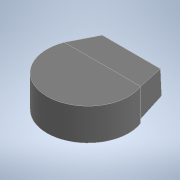
# Autodesk Inventor part: vez-nova
Saved by Autodesk Inventor 2022 (Build 260153000, 153)
## iProperties
Created: 2022-12-19
Part Number: vez-nova
Material: Generic
Document SubType Name: Modeling
Designer: matys
Density: 1 g/cm^3
Appearance: Gray
Author: matys
Autodesk Inventor part; units mm, degrees
ref_plane "YZ Plane" through (0, 0, 0) normal (1, 0, 0) x (0, 1, 0)
ref_plane "XZ Plane" through (0, 0, 0) normal (0, 1, 0) x (-1, 0, 0)
ref_plane "XY Plane" through (0, 0, 0) normal (0, 0, 1) x (1, 0, 0)
sketch "Sketch1" plane through (0, 0, 0) normal (0, 1, 0) x (-1, 0, 0)
  arc A0 (46.7052, -17.85) -> (-46.7052, -17.85) centre (0, 0) ccw
  line L0 (0, 0) -> (0, -55.2)
  line L1 (0, -55.2) -> (35, -55.2)
  line L2 (0, -55.2) -> (-35, -55.2)
  line L3 (0, 50) -> (0, -17.85)
  line L4 (0, -17.85) -> (46.7052, -17.85)
  line L5 (0, -17.85) -> (-46.7052, -17.85)
  line L6 (-46.7052, -17.85) -> (-35, -55.2)
  line L7 (46.7052, -17.85) -> (35, -55.2)
  line L8 (35, -55.2) -> (33, -55.2)
  line L9 (-35, -55.2) -> (-33, -55.2)
  line L10 (0, 50) -> (0, 48)
  arc A1 (44.5576, -17.85) -> (-44.5576, -17.85) centre (0, 0) ccw
  line L11 (44.5576, -17.85) -> (33, -55.2)
  line L12 (-44.5576, -17.85) -> (-33, -55.2)
  dimension "d0" = 100
  dimension "d4" = 55.2
  dimension "d5" = 35
  dimension "d6" = 67.85
  dimension "d7" = 2
  dimension "d8" = 2
  dimension "d9" = 2
  constraints: 26 end point, 7 point on line, 6 point on circle, 3 coincident, 2 centre point, 1 horizontal, 1 perpendicular
  measures "d0" diameter of A0
  measures "d4" distance of L0.start L0.end
  measures "d5" distance of L0.end L2.end
  measures "d6" distance of L3.start L3.end
  measures "d7" distance of L1.end L8.end
  measures "d8" distance of L2.end L9.end
  measures "d9" distance of L3.start L10.end
extrude "Extrusion1" add sketch "Sketch1" along normal blind 34.5
chamfer "Chamfer3" distance 2.3 distance2 34.5 2 edges at (-17.5, 34.5, -55.2) (17.5, 34.5, -55.2) measured on face at (-17.5, 34.5, -54.7) measured on face at (17.5, 34.5, -54.7)
chamfer "Chamfer4" distance 4.6 distance2 35.05 2 edges at (-17.8604, 34.5, -52.9001) (17.8604, 34.5, -52.9001) measured on face at (17.8604, 34.0011, -52.9334) measured on face at (-17.8604, 34.0011, -52.9334)
sketch "Sketch3" plane through (0, 0, 0) normal (0, -1, 0) x (1, 0, 0)
  line L0 (0, 0) -> (0, 34.5)
  circle A0 centre (0, 0) radius 34.5
  circle A1 centre (0, 0) radius 36.8
  circle A2 centre (0, 0) radius 37.375
  line L1 (0, -36.8) -> (0, -41.4)
  line L2 (0, -41.4) -> (17.5375, -41.4)
  line L3 (0, -41.4) -> (-17.5375, -41.4)
  arc A3 (46.7052, -17.85) -> (-46.7052, -17.85) centre (0, 0) ccw
  line L4 (46.7052, -17.85) -> (35, -55.2) projected
  line L5 (46.7052, -17.85) -> (17.5375, -41.4)
  arc A4 (46.7052, -17.85) -> (-46.7052, -17.85) centre (0, 0) ccw projected
  line L6 (-46.7052, -17.85) -> (-17.5375, -41.4)
  dimension "d25" = 73.6
  dimension "d24" = 34.5
  dimension "d26" = 74.75
  dimension "d27" = 4.6
  dimension "d28" = 17.5375
  constraints: 12 end point, 4 coincident, 2 centre point, 2 point on circle, 2 vertical, 2 vertical alignment, 1 horizontal, 1 symmetric about line, 4 other
  measures "d24" distance of L0.start L0.end
  measures "d26" diameter of A2
  measures "d27" distance of L1.start L1.end
  measures "d28" distance of L1.end L2.end
extrude "Extrusion2" add sketch "Sketch3" along normal blind 4.6 contours A0 | A1 | A2 | L3 L6 A3 L5 L2
sketch "Sketch4" plane through (0, -4.6, 0) normal (0, -1, 0) x (1, 0, 0)
  line L0 (0, 0) -> (0, -34.5)
  circle A0 centre (0, 0) radius 34.5
  line L1 (0, -34.5) -> (0, -37)
  circle A1 centre (0, 0) radius 37
  dimension "d31" = 34.5
  dimension "d32" = 2.5
  constraints: 4 end point, 2 coincident, 2 vertical, 2 vertical alignment, 4 other
  measures "d31" distance of L0.start L0.end
  measures "d32" distance of L0.end L1.end
extrude "Extrusion3" add sketch "Sketch4" along normal blind 5.75
sketch "Sketch5" plane through (0, -4.6, 0) normal (0, -1, 0) x (1, 0, 0)
  circle A0 centre (0, 0) radius 30.8955
  circle A1 centre (0, 0) radius 30
  dimension "d62" = 60
  constraints: 2 centre point, 2 coincident
  measures "d62" diameter of A1
extrude "Extrusion4" cut sketch "Sketch5" against normal blind 34.5 contours A1
sketch "Sketch6" plane through (0, -10.35, 0) normal (0, -1, 0) x (1, 0, 0)
  circle A0 centre (0, 0) radius 37
  constraints: 1 centre point, 1 coincident
extrude "Extrusion5" cut sketch "Sketch6" against normal blind 5.75
sketch "Sketch7" plane through (0, -4.6, 0) normal (0, -1, 0) x (1, 0, 0)
  line L0 (17.5375, -41.4) -> (-17.5375, -41.4) projected
  circle A0 centre (0, 0) radius 33.6
  circle A1 centre (0, 0) radius 30.0896
  dimension "d61" = 67.2
  constraints: 2 centre point, 1 coincident
  measures "d61" diameter of A0
extrude "Extrusion6" cut sketch "Sketch7" against normal blind 5.75 contours A0 | A1
sketch "Sketch8" plane through (0, 1.15, 0) normal (0, -1, 0) x (1, 0, 0)
  circle A0 centre (0, 0) radius 34.3955 projected
  line L0 (34.3955, 0) -> (-34.3955, 0)
  line L1 (41.6045, -3) -> (-34.3955, -3)
  line L2 (41.6045, 3) -> (-34.3955, 3)
  circle A1 centre (0, 0) radius 34.5
  circle A2 centre (0, 0) radius 34.3955
  circle A3 centre (0, 0) radius 30
  circle A4 centre (0, 0) radius 33.6
  point P0 (-34.3693, -3)
  point P1 (-34.3693, 3)
  point P2 (-34.2644, 3)
  point P3 (-34.2644, -3)
  point P4 (34.3693, -3)
  point P5 (34.2644, -3)
  point P6 (34.2644, 3)
  point P7 (34.3693, 3)
  point P8 (29.8496, -3)
  point P9 (29.8496, 3)
  point P10 (-29.8496, -3)
  point P11 (-29.8496, 3)
  point P12 (-33.4658, 3)
  point P13 (-33.4658, -3)
  point P14 (33.4658, -3)
  point P15 (33.4658, 3)
  dimension "d42" = 3
  dimension "d43" = 3
  constraints: 6 end point, 3 centre point, 3 coincident, 2 parallel, 2 point on circle, 1 horizontal, 1 horizontal alignment, 2 other
  measures "d42" distance between parallel lines of L0 L1
  measures "d43" distance between parallel lines of L0 L2
extrude "Extrusion7" cut sketch "Sketch8" against normal blind 5.75 contours A4 L1 A3 L0 | L0 A3 L2 A4 | L2 A3 L0 A4 | A4 L0 A3 L1
ref_plane "Work Plane1" through (8.75, 34.5, -17.85) normal (0, 0, 1) x (1, 0, 0)
sketch "Sketch9" plane through (8.75, 34.5, -17.85) normal (0, 0, 1) x (1, 0, 0)
  line L0 (37.9552, 0) -> (26.8749, -4.5898) projected
  line L1 (26.8749, -4.5898) -> (26.1514, -34.5)
  line L2 (37.9552, -34.5) -> (8.7875, -34.5) projected
  line L3 (-43.75, -34.5) -> (-44.3749, -4.5898) projected
  line L4 (-43.75, -34.5) -> (-40.75, -34.5)
  line L5 (-26.2875, -34.5) -> (-55.4552, -34.5) projected
  line L6 (-40.75, -34.5) -> (-40.75, -31.5)
  line L7 (-40.75, -31.5) -> (-40.75, -4.5898)
  line L8 (-40.75, -4.5898) -> (-40.75, -7.5898)
  line L9 (-40.75, -7.5898) -> (-40.75, -31.5)
  line L10 (25.75, -27.6) -> (25.75, -4.6) projected
  line L11 (26.8749, -4.5898) -> (26.25, -34.5) projected
  line L12 (26.25, -34.5) -> (23.25, -34.5)
  line L13 (23.25, -34.5) -> (23.25, -31.5)
  line L14 (23.25, -31.5) -> (-40.75, -31.5)
  line L15 (23.25, -31.5) -> (23.25, -7.5898)
  line L16 (23.25, -7.5898) -> (-40.75, -7.5898)
  point P0 (-8.75, -34.5)
  dimension "d46" = 3
  dimension "d47" = 3
  dimension "d48" = 3
  dimension "d49" = 3
  dimension "d50" = 3
  constraints: 22 end point, 6 point on line, 3 perpendicular, 1 parallel
  measures "d46" distance of L3.start L4.end
  measures "d47" distance of L4.end L6.end
  measures "d48" distance of L7.end L8.end
  measures "d49" distance of L11.end L12.end
  measures "d50" distance of L12.end L13.end
extrude "Extrusion8" cut sketch "Sketch9" along normal blind 10 and the other way blind 100 contours L7 L16 L15 L14
sketch "Sketch10" plane through (32, 3, -12.8938) normal (-1, 0, 0) x (0, 0, 1)
  line L0 (-42.1062, 0) -> (-40.5122, 23.9102)
  line L1 (-40.5122, 23.9102) -> (-41.3092, 11.9551)
  line L2 (-42.1062, 0) -> (-40.5122, 23.9102) projected
  line L3 (-41.3092, 11.9551) -> (-31.3092, 11.9551)
  line L4 (-31.3092, 11.9551) -> (-35.8092, 11.9551)
  circle A0 centre (-31.3092, 11.9551) radius 4.5
  point P0 (12.8938, -3)
  dimension "d55" = 10
  dimension "d56" = 4.5
  constraints: 8 end point, 1 coincident, 1 horizontal, 1 horizontal alignment, 1 midpoint, 1 point on line, 2 other
  measures "d55" distance of L1.end L3.end
  measures "d56" distance of L3.end L4.end
extrude "Extrusion9" cut sketch "Sketch10" along normal blind 66 and the other way blind 2
sketch "Sketch13" plane through (0, 29.9, 0) normal (0, -1, 0) x (1, 0, 0)
  line L0 (0, 0) -> (5.6, 0)
  line L1 (5.6, 0) -> (5.6, -5.6)
  line L2 (5.6, -5.6) -> (-5.6, -5.6)
  line L3 (-5.6, -5.6) -> (-5.6, 5.6)
  line L4 (-5.6, 5.6) -> (5.6, 5.6)
  line L5 (5.6, 5.6) -> (5.6, 0)
  dimension "d64" = 5.6
  dimension "d65" = 5.6
  dimension "d66" = 11.2
  dimension "d67" = 11.2
  constraints: 12 end point, 4 perpendicular, 1 horizontal, 1 vertical
  measures "d64" distance of L0.start L0.end
  measures "d65" distance of L0.end L1.end
  measures "d66" distance of L1.end L2.end
  measures "d67" distance of L2.end L3.end
extrude "Extrusion10" cut sketch "Sketch13" against normal blind 2.5
sketch "Sketch14" plane through (0, 29.9, 0) normal (0, -1, 0) x (1, 0, 0)
  line L0 (5.6, -5.6) -> (-5.6, -5.6) projected
  line L1 (5.6, 5.6) -> (5.6, -5.6) projected
  line L2 (-5.6, -5.6) -> (5.6, -5.6)
  line L3 (5.6, -5.6) -> (5.6, 5.6)
  line L4 (5.6, 5.6) -> (-5.6, 5.6)
  line L5 (-5.6, 5.6) -> (-5.6, -5.6)
  line L6 (-5.6, -5.6) -> (-5.6, 5.6) projected
  line L7 (-5.6, 0) -> (-8.6, 0)
  line L8 (-5.6, 5.6) -> (5.6, 5.6) projected
  line L9 (0, 5.6) -> (0, 8.6)
  line L10 (0, 8.6) -> (-8.6, 8.6)
  line L11 (-8.6, 8.6) -> (-8.6, 0)
  line L12 (5.6, 0) -> (8.6, 0)
  line L13 (8.6, 0) -> (8.6, 8.6)
  line L14 (8.6, 8.6) -> (0, 8.6)
  line L15 (0, -5.6) -> (0, -8.6)
  line L16 (0, -8.6) -> (-8.6, -8.6)
  line L17 (-8.6, -8.6) -> (-8.6, 0)
  line L18 (0, -8.6) -> (8.6, -8.6)
  line L19 (8.6, 0) -> (8.6, -8.6)
  point P0 (0, 0)
  dimension "d70" = 3
  dimension "d71" = 3
  dimension "d72" = 3
  dimension "d73" = 3
  constraints: 32 end point, 8 perpendicular, 5 point on line, 4 midpoint, 3 horizontal, 2 parallel, 1 vertical
  measures "d70" distance of L7.start L7.end
  measures "d71" distance of L9.start L9.end
  measures "d72" distance of L12.start L12.end
  measures "d73" distance of L15.start L15.end
extrude "Extrusion11" add sketch "Sketch14" along normal blind 10 contours L1 L12 L19 L18 L15 L0 | L15 L16 L17 L7 L5 L0 | L1 L4 L9 L14 L13 L12 | L7 L11 L10 L9 L4 L5
body "Solid1"
